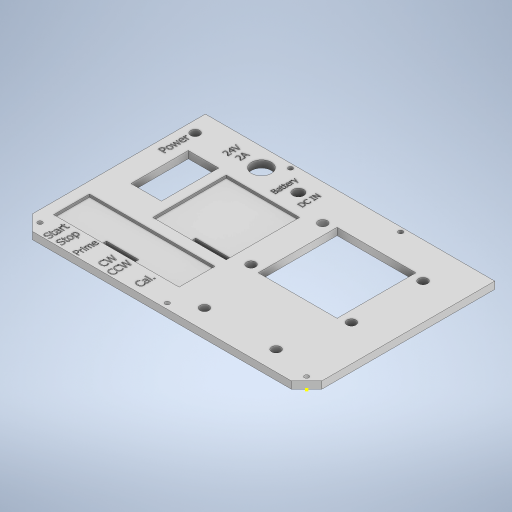
# Autodesk Inventor part: Ele Panel
Saved by Autodesk Inventor 2023 (Build 270158000, 158)
## iProperties
Created: 2023-08-23
Part Number: Ele Panel
Material: Generic
Document SubType Name: Modeling
Designer: alian
Density: 1 g/cm^3
Appearance: Default
Author: alian
Autodesk Inventor part; units mm, degrees
(part 1 of 2)
ref_plane "YZ Plane" through (0, 0, 0) normal (1, 0, 0) x (0, 1, 0)
ref_plane "XZ Plane" through (0, 0, 0) normal (0, 1, 0) x (-1, 0, 0)
ref_plane "XY Plane" through (0, 0, 0) normal (0, 0, 1) x (1, 0, 0)
sketch "Sketch1" plane through (0, 0, 0) normal (0, 1, 0) x (-1, 0, 0)
  line L0 (0, 0) -> (161.5, 0)
  line L1 (161.5, 0) -> (161.5, -105)
  line L2 (161.5, -105) -> (0, -105)
  line L3 (0, -105) -> (0, 0)
  dimension "d0" = 161.5
  dimension "d1" = 105
  constraints: 8 end point, 2 parallel, 1 horizontal, 1 perpendicular
  measures "d0" distance of L1.end L2.end
  measures "d1" distance of L0.end L1.end
extrude "Extrusion1" add sketch "Sketch1" along normal blind 4
sketch "Sketch2" plane through (0, 4, 0) normal (0, 1, 0) x (1, 0, 0)
  line L0 (-148.6423, 50.601) -> (-131.6423, 50.601)
  line L1 (-131.6423, 50.601) -> (-131.6423, 82.601)
  line L2 (-131.6423, 82.601) -> (-148.6423, 82.601)
  line L3 (-148.6423, 82.601) -> (-148.6423, 50.601)
  circle A0 centre (-148.9719, 88.0693) radius 1.5
  circle A1 centre (-131.2982, 88.0693) radius 1.5
  circle A2 centre (-131.2982, 42.7853) radius 1.5
  circle A3 centre (-148.9719, 42.7853) radius 1.5
  line L4 (-141.2539, 141.0846) -> (-141.2539, 196.4251) construction
  line L5 (-141.2539, 196.4251) -> (-113.1686, 196.4251) construction
  line L6 (-113.1686, 196.4251) -> (-113.1686, 141.0846) construction
  line L7 (-113.1686, 141.0846) -> (-141.2539, 141.0846) construction
  line L8 (-173.7219, 134.419) -> (-150.8919, 134.419)
  line L9 (-150.8919, 134.419) -> (-150.8919, 185.551)
  line L10 (-150.8919, 185.551) -> (-173.7219, 185.551)
  line L11 (-173.7219, 185.551) -> (-173.7219, 134.419)
  line L12 (-155.1907, 14) -> (-85.1907, 14)
  line L13 (-85.1907, 14) -> (-85.1907, 34)
  line L14 (-85.1907, 34) -> (-155.1907, 34)
  line L15 (-155.1907, 34) -> (-155.1907, 14)
  line L16 (-126.1907, 40.3041) -> (-85.1907, 40.3041)
  line L17 (-85.1907, 40.3041) -> (-85.1907, 81.3041)
  line L18 (-85.1907, 81.3041) -> (-126.1907, 81.3041)
  line L19 (-126.1907, 81.3041) -> (-126.1907, 40.3041)
  line L20 (-84, 33) -> (-12, 33)
  line L21 (-12, 33) -> (-12, 100)
  line L22 (-12, 100) -> (-84, 100)
  line L23 (-84, 100) -> (-84, 33)
  circle A4 centre (-68, 11) radius 2.5
  circle A5 centre (-28, 11) radius 2.5
  circle A6 centre (-119.8496, 94.6341) radius 5.5
  circle A7 centre (-97.5813, 93) radius 3
  circle A8 centre (-155.1907, 93) radius 2.5
  circle A9 centre (-88.5813, 93) radius 2.55
  line L24 (0, 105) -> (-161.5, 105) projected
  line L25 (0, 0) -> (0, 105) projected
  line L26 (-161.5, 0) -> (0, 0) projected
  line L27 (-70, 43) -> (-26, 43)
  line L28 (-26, 43) -> (-26, 87)
  line L29 (-26, 87) -> (-70, 87)
  line L30 (-70, 87) -> (-70, 43)
  point P0 (-120.1907, 14)
  point P1 (-48, 43)
  dimension "d4" = 17
  dimension "d5" = 32
  dimension "d12" = 22.83
  dimension "d13" = 51.132
  dimension "d30" = 3
  dimension "d39" = 7.8157
  dimension "d40" = 0.3296
  dimension "d42" = 0.344
  dimension "d44" = 5.4682
  dimension "d47" = 70
  dimension "d48" = 20
  dimension "d50" = 41
  dimension "d51" = 41
  dimension "d53" = 72
  dimension "d54" = 67
  dimension "d56" = 5
  dimension "d57" = 5
  dimension "d58" = 16
  dimension "d59" = 16
  dimension "d60" = 22
  dimension "d68" = 11
  dimension "d71" = 6
  dimension "d74" = 5
  dimension "d75" = 5.1
  dimension "d76" = 9
  dimension "d132" = 5
  dimension "d133" = 12
  dimension "d155" = 12
  dimension "d156" = 14
  dimension "d157" = 44
  dimension "d158" = 44
  dimension "d159" = 14
  dimension "d161" = 10
  constraints: 48 end point, 12 parallel, 10 centre point, 6 horizontal, 6 perpendicular, 5 horizontal alignment, 3 equal radius, 3 vertical alignment, 2 midpoint, 2 other
  measures "d4" distance of L2.end L1.end
  measures "d5" distance of L1.end L0.end
  measures "d12" distance of L10.end L9.end
  measures "d13" distance of L9.end L8.end
  measures "d30" diameter of A0
  measures "d39" distance from line of L0 A3.centre
  measures "d40" distance from line of A3.centre L3
  measures "d42" distance from line of L1 A2.centre
  measures "d44" distance from line of A0.centre L2
  measures "d47" distance of L14.end L13.end
  measures "d48" distance of L13.end L12.end
  measures "d50" distance of L18.end L17.end
  measures "d51" distance of L17.end L16.end
  measures "d53" distance of L22.end L21.end
  measures "d54" distance of L21.end L20.end
  measures "d56" diameter of A4
  measures "d57" diameter of A5
  measures "d58" distance from line of L23 A4.centre
  measures "d59" distance from line of L21 A5.centre
  measures "d60" distance from line of L20 A4.centre
  measures "d68" diameter of A6
  measures "d71" diameter of A7
  measures "d74" diameter of A8
  measures "d75" diameter of A9
  measures "d76" distance of A7.centre A9.centre
  measures "d132" distance between parallel lines of L24 L22
  measures "d133" distance between parallel lines of L21 L25
  measures "d155" distance from line of L24 A7.centre
  measures "d156" distance from line of L26 point (-120.191, 14)
  measures "d157" distance from line of L29 point (-48, 43)
  measures "d158" distance between parallel lines of L28 L30
  measures "d159" distance between parallel lines of L23 L30
  measures "d161" distance between parallel lines of L20 L27
extrude "Extrusion2" cut sketch "Sketch2" against normal blind 4 contours L3 L2 L1 L0 | A4 | A5 | A6 | A7 | A8 | L30 L29 L28 L27
sketch "Sketch3" plane through (0, 4, 0) normal (0, 1, 0) x (1, 0, 0)
  line L0 (-106.2715, 85.6469) -> (-106.2715, 98.9463) construction
  line L1 (-106.2715, 98.9463) -> (-102.5043, 98.9463) construction
  line L2 (-102.5043, 98.9463) -> (-102.5043, 85.6469) construction
  line L3 (-102.5043, 85.6469) -> (-106.2715, 85.6469) construction
  line L4 (-92.3295, 86.7189) -> (-92.3295, 97.75) construction
  line L5 (-92.3295, 97.75) -> (-89.0807, 97.75) construction
  line L6 (-89.0807, 97.75) -> (-89.0807, 86.7189) construction
  line L7 (-89.0807, 86.7189) -> (-92.3295, 86.7189) construction
  line L8 (-138.4009, 85.1047) -> (-138.4009, 104.5309) construction
  line L9 (-138.4009, 104.5309) -> (-128.5308, 104.5309) construction
  line L10 (-128.5308, 104.5309) -> (-128.5308, 85.1047) construction
  line L11 (-128.5308, 85.1047) -> (-138.4009, 85.1047) construction
  line L12 (-148.6469, 2.1995) -> (-148.6469, 11.1409) construction
  line L13 (-148.6469, 11.1409) -> (-144.6208, 11.1409) construction
  line L14 (-144.6208, 11.1409) -> (-144.6208, 2.1995) construction
  line L15 (-144.6208, 2.1995) -> (-148.6469, 2.1995) construction
  line L16 (-132.0468, 0.8832) -> (-132.0468, 11.3907) construction
  line L17 (-132.0468, 11.3907) -> (-128.9272, 11.3907) construction
  line L18 (-128.9272, 11.3907) -> (-128.9272, 0.8832) construction
  line L19 (-128.9272, 0.8832) -> (-132.0468, 0.8832) construction
  line L20 (-119.8791, 2.3194) -> (-119.8791, 11.1324) construction
  line L21 (-119.8791, 11.1324) -> (-111.7039, 11.1324) construction
  line L22 (-111.7039, 11.1324) -> (-111.7039, 2.3194) construction
  line L23 (-111.7039, 2.3194) -> (-119.8791, 2.3194) construction
  line L24 (-100.0402, 3.0337) -> (-100.0402, 9.9794) construction
  line L25 (-100.0402, 9.9794) -> (-92.1934, 9.9794) construction
  line L26 (-92.1934, 9.9794) -> (-92.1934, 3.0337) construction
  line L27 (-92.1934, 3.0337) -> (-100.0402, 3.0337) construction
  line L28 (-157.8178, 74.3524) -> (-157.8178, 89.3313) construction
  line L29 (-157.8178, 89.3313) -> (-153.7335, 89.3313) construction
  line L30 (-153.7335, 89.3313) -> (-153.7335, 74.3524) construction
  line L31 (-153.7335, 74.3524) -> (-157.8178, 74.3524) construction
  spline S0 degree 2 poles (-95.7906, 5.0013) (-95.7906, 4.6123) (-96.0532, 3.9543) (-96.3158, 3.7144) knots 0 0 0 1 2 2 2
  spline S1 degree 2 poles (-96.3158, 3.7144) (-96.5751, 3.4745) (-97.353, 3.212) (-97.8587, 3.212) knots 0 0 0 1 2 2 2
  spline S2 degree 2 poles (-97.8587, 3.212) (-98.3611, 3.212) (-99.1067, 3.4681) (-99.3822, 3.7112) knots 0 0 0 1 2 2 2
  spline S3 degree 2 poles (-99.3822, 3.7112) (-99.6513, 3.951) (-99.9333, 4.6058) (-99.9333, 5.011) knots 0 0 0 1 2 2 2
  spline S4 degree 2 poles (-99.9333, 5.011) (-99.9333, 5.212) (-99.8749, 5.5653) (-99.8295, 5.7144) knots 0 0 0 1 2 2 2
  spline S5 degree 2 poles (-99.8295, 5.7144) (-99.7874, 5.8441) (-99.6675, 6.1131) (-99.5962, 6.246) knots 0 0 0 1 2 2 2
  line L32 (-99.5962, 6.246) -> (-98.9543, 6.246)
  line L33 (-98.9543, 6.246) -> (-98.9543, 6.2039)
  spline S6 degree 2 poles (-98.9543, 6.2039) (-99.0192, 6.1326) (-99.2007, 5.9121) (-99.2882, 5.7533) knots 0 0 0 1 2 2 2
  spline S7 degree 2 poles (-99.2882, 5.7533) (-99.3725, 5.601) (-99.4795, 5.2412) (-99.4795, 5.0078) knots 0 0 0 1 2 2 2
  spline S8 degree 2 poles (-99.4795, 5.0078) (-99.4795, 4.7517) (-99.2688, 4.2946) (-99.0678, 4.1228) knots 0 0 0 1 2 2 2
  spline S9 degree 2 poles (-99.0678, 4.1228) (-98.8636, 3.9543) (-98.2445, 3.7663) (-97.8587, 3.7663) knots 0 0 0 1 2 2 2
  spline S10 degree 2 poles (-97.8587, 3.7663) (-97.447, 3.7663) (-96.8539, 3.964) (-96.6496, 4.1358) knots 0 0 0 1 2 2 2
  spline S11 degree 2 poles (-96.6496, 4.1358) (-96.4519, 4.3044) (-96.2509, 4.7549) (-96.2509, 5.0078) knots 0 0 0 1 2 2 2
  spline S12 degree 2 poles (-96.2509, 5.0078) (-96.2509, 5.2379) (-96.3644, 5.6301) (-96.4487, 5.7825) knots 0 0 0 1 2 2 2
  spline S13 degree 2 poles (-96.4487, 5.7825) (-96.5329, 5.9283) (-96.708, 6.1455) (-96.7696, 6.2071) knots 0 0 0 1 2 2 2
  line L34 (-96.7696, 6.2071) -> (-96.7696, 6.246)
  line L35 (-96.7696, 6.246) -> (-96.1342, 6.246)
  spline S14 degree 2 poles (-96.1342, 6.246) (-96.0727, 6.1131) (-95.9592, 5.8797) (-95.9073, 5.7144) knots 0 0 0 1 2 2 2
  spline S15 degree 2 poles (-95.9073, 5.7144) (-95.849, 5.5394) (-95.7906, 5.2412) (-95.7906, 5.0013) knots 0 0 0 1 2 2 2
  spline S16 degree 2 poles (-96.1796, 8.3757) (-96.1342, 8.3141) (-95.9722, 8.1066) (-95.9235, 8.0094) knots 0 0 0 1 2 2 2
  spline S17 degree 2 poles (-95.9235, 8.0094) (-95.8522, 7.8765) (-95.7777, 7.6269) (-95.7777, 7.4) knots 0 0 0 1 2 2 2
  spline S18 degree 2 poles (-95.7777, 7.4) (-95.7777, 7.2152) (-95.9171, 6.8813) (-96.0435, 6.7549) knots 0 0 0 1 2 2 2
  spline S19 degree 2 poles (-96.0435, 6.7549) (-96.1667, 6.635) (-96.5297, 6.4891) (-96.7307, 6.4891) knots 0 0 0 1 2 2 2
  spline S20 degree 2 poles (-96.7307, 6.4891) (-97.0419, 6.4891) (-97.4827, 6.7517) (-97.6091, 7.0369) knots 0 0 0 1 2 2 2
  spline S21 degree 2 poles (-97.6091, 7.0369) (-97.7258, 7.2898) (-97.8133, 7.977) (-97.836, 8.3757) knots 0 0 0 1 2 2 2
  line L36 (-97.836, 8.3757) -> (-97.9333, 8.3757)
  spline S22 degree 2 poles (-97.9333, 8.3757) (-98.1083, 8.3757) (-98.3255, 8.2687) (-98.3871, 8.1715) knots 0 0 0 1 2 2 2
  spline S23 degree 2 poles (-98.3871, 8.1715) (-98.4487, 8.0742) (-98.4876, 7.7954) (-98.4876, 7.6463) knots 0 0 0 1 2 2 2
  spline S24 degree 2 poles (-98.4876, 7.6463) (-98.4876, 7.4713) (-98.3838, 6.998) (-98.2833, 6.7614) knots 0 0 0 1 2 2 2
  line L37 (-98.2833, 6.7614) -> (-98.2833, 6.7322)
  line L38 (-98.2833, 6.7322) -> (-98.7987, 6.7322)
  spline S25 degree 2 poles (-98.7987, 6.7322) (-98.8376, 6.8716) (-98.9349, 7.3935) (-98.9349, 7.6496) knots 0 0 0 1 2 2 2
  spline S26 degree 2 poles (-98.9349, 7.6496) (-98.9349, 7.9608) (-98.8376, 8.3854) (-98.7112, 8.554) knots 0 0 0 1 2 2 2
  spline S27 degree 2 poles (-98.7112, 8.554) (-98.588, 8.7193) (-98.1958, 8.8813) (-97.9138, 8.8813) knots 0 0 0 1 2 2 2
  line L39 (-97.9138, 8.8813) -> (-95.862, 8.8813)
  line L40 (-95.862, 8.8813) -> (-95.862, 8.3757)
  line L41 (-95.862, 8.3757) -> (-96.1796, 8.3757)
  line L42 (-96.601, 8.3757) -> (-97.4341, 8.3757)
  spline S28 degree 2 poles (-97.4341, 8.3757) (-97.4179, 8.1942) (-97.3628, 7.6463) (-97.3109, 7.4745) knots 0 0 0 1 2 2 2
  spline S29 degree 2 poles (-97.3109, 7.4745) (-97.2493, 7.2736) (-96.9932, 7.011) (-96.7663, 7.011) knots 0 0 0 1 2 2 2
  spline S30 degree 2 poles (-96.7663, 7.011) (-96.507, 7.011) (-96.2445, 7.3027) (-96.2445, 7.5815) knots 0 0 0 1 2 2 2
  spline S31 degree 2 poles (-96.2445, 7.5815) (-96.2445, 7.8181) (-96.4487, 8.2071) (-96.601, 8.3757) knots 0 0 0 1 2 2 2
  line L43 (-95.862, 10.1066) -> (-95.862, 9.601)
  line L44 (-95.862, 9.601) -> (-100.0402, 9.601)
  line L45 (-100.0402, 9.601) -> (-100.0402, 10.1066)
  line L46 (-100.0402, 10.1066) -> (-95.862, 10.1066)
  line L47 (-95.862, 11.6334) -> (-95.862, 10.9916)
  line L48 (-95.862, 10.9916) -> (-96.6269, 10.9916)
  line L49 (-96.6269, 10.9916) -> (-96.6269, 11.6334)
  line L50 (-96.6269, 11.6334) -> (-95.862, 11.6334)
  spline S32 degree 2 poles (-115.7364, 4.5622) (-115.7364, 4.1732) (-115.999, 3.5152) (-116.2616, 3.2753) knots 0 0 0 1 2 2 2
  spline S33 degree 2 poles (-116.2616, 3.2753) (-116.5209, 3.0354) (-117.2988, 2.7729) (-117.8045, 2.7729) knots 0 0 0 1 2 2 2
  spline S34 degree 2 poles (-117.8045, 2.7729) (-118.3069, 2.7729) (-119.0525, 3.029) (-119.328, 3.2721) knots 0 0 0 1 2 2 2
  spline S35 degree 2 poles (-119.328, 3.2721) (-119.5971, 3.5119) (-119.8791, 4.1667) (-119.8791, 4.5719) knots 0 0 0 1 2 2 2
  spline S36 degree 2 poles (-119.8791, 4.5719) (-119.8791, 4.7729) (-119.8207, 5.1262) (-119.7753, 5.2753) knots 0 0 0 1 2 2 2
  spline S37 degree 2 poles (-119.7753, 5.2753) (-119.7332, 5.405) (-119.6133, 5.674) (-119.542, 5.8069) knots 0 0 0 1 2 2 2
  line L51 (-119.542, 5.8069) -> (-118.9001, 5.8069)
  line L52 (-118.9001, 5.8069) -> (-118.9001, 5.7648)
  spline S38 degree 2 poles (-118.9001, 5.7648) (-118.965, 5.6935) (-119.1465, 5.473) (-119.234, 5.3142) knots 0 0 0 1 2 2 2
  spline S39 degree 2 poles (-119.234, 5.3142) (-119.3183, 5.1619) (-119.4253, 4.8021) (-119.4253, 4.5687) knots 0 0 0 1 2 2 2
  spline S40 degree 2 poles (-119.4253, 4.5687) (-119.4253, 4.3126) (-119.2146, 3.8555) (-119.0136, 3.6837) knots 0 0 0 1 2 2 2
  spline S41 degree 2 poles (-119.0136, 3.6837) (-118.8094, 3.5152) (-118.1902, 3.3272) (-117.8045, 3.3272) knots 0 0 0 1 2 2 2
  spline S42 degree 2 poles (-117.8045, 3.3272) (-117.3928, 3.3272) (-116.7996, 3.5249) (-116.5954, 3.6967) knots 0 0 0 1 2 2 2
  spline S43 degree 2 poles (-116.5954, 3.6967) (-116.3977, 3.8653) (-116.1967, 4.3158) (-116.1967, 4.5687) knots 0 0 0 1 2 2 2
  spline S44 degree 2 poles (-116.1967, 4.5687) (-116.1967, 4.7988) (-116.3102, 5.191) (-116.3945, 5.3434) knots 0 0 0 1 2 2 2
  spline S45 degree 2 poles (-116.3945, 5.3434) (-116.4787, 5.4893) (-116.6538, 5.7064) (-116.7154, 5.768) knots 0 0 0 1 2 2 2
  line L53 (-116.7154, 5.768) -> (-116.7154, 5.8069)
  line L54 (-116.7154, 5.8069) -> (-116.08, 5.8069)
  spline S46 degree 2 poles (-116.08, 5.8069) (-116.0184, 5.674) (-115.905, 5.4406) (-115.8531, 5.2753) knots 0 0 0 1 2 2 2
  spline S47 degree 2 poles (-115.8531, 5.2753) (-115.7948, 5.1003) (-115.7364, 4.8021) (-115.7364, 4.5622) knots 0 0 0 1 2 2 2
  line L55 (-119.8078, 10.7858) -> (-115.8078, 9.781)
  line L56 (-115.8078, 9.781) -> (-115.8078, 9.1846)
  line L57 (-115.8078, 9.1846) -> (-119.127, 8.3709)
  line L58 (-119.127, 8.3709) -> (-115.8078, 7.58)
  line L59 (-115.8078, 7.58) -> (-115.8078, 6.9901)
  line L60 (-115.8078, 6.9901) -> (-119.8078, 5.969)
  line L61 (-119.8078, 5.969) -> (-119.8078, 6.5168)
  line L62 (-119.8078, 6.5168) -> (-116.4917, 7.3207)
  line L63 (-116.4917, 7.3207) -> (-119.8078, 8.1181)
  line L64 (-119.8078, 8.1181) -> (-119.8078, 8.6594)
  line L65 (-119.8078, 8.6594) -> (-116.4528, 9.4633)
  line L66 (-116.4528, 9.4633) -> (-119.8078, 10.264)
  line L67 (-119.8078, 10.264) -> (-119.8078, 10.7858)
  spline S48 degree 2 poles (-109.1505, 2.9106) (-109.1505, 2.5217) (-109.4131, 1.8636) (-109.6757, 1.6238) knots 0 0 0 1 2 2 2
  spline S49 degree 2 poles (-109.6757, 1.6238) (-109.935, 1.3839) (-110.7129, 1.1213) (-111.2186, 1.1213) knots 0 0 0 1 2 2 2
  spline S50 degree 2 poles (-111.2186, 1.1213) (-111.721, 1.1213) (-112.4666, 1.3774) (-112.7421, 1.6205) knots 0 0 0 1 2 2 2
  spline S51 degree 2 poles (-112.7421, 1.6205) (-113.0112, 1.8604) (-113.2932, 2.5152) (-113.2932, 2.9204) knots 0 0 0 1 2 2 2
  spline S52 degree 2 poles (-113.2932, 2.9204) (-113.2932, 3.1213) (-113.2348, 3.4747) (-113.1894, 3.6238) knots 0 0 0 1 2 2 2
  spline S53 degree 2 poles (-113.1894, 3.6238) (-113.1473, 3.7534) (-113.0274, 4.0225) (-112.9561, 4.1554) knots 0 0 0 1 2 2 2
  line L68 (-112.9561, 4.1554) -> (-112.3142, 4.1554)
  line L69 (-112.3142, 4.1554) -> (-112.3142, 4.1132)
  spline S54 degree 2 poles (-112.3142, 4.1132) (-112.3791, 4.0419) (-112.5606, 3.8215) (-112.6481, 3.6627) knots 0 0 0 1 2 2 2
  spline S55 degree 2 poles (-112.6481, 3.6627) (-112.7324, 3.5103) (-112.8394, 3.1505) (-112.8394, 2.9171) knots 0 0 0 1 2 2 2
  spline S56 degree 2 poles (-112.8394, 2.9171) (-112.8394, 2.6611) (-112.6287, 2.204) (-112.4277, 2.0322) knots 0 0 0 1 2 2 2
  spline S57 degree 2 poles (-112.4277, 2.0322) (-112.2235, 1.8636) (-111.6044, 1.6756) (-111.2186, 1.6756) knots 0 0 0 1 2 2 2
  spline S58 degree 2 poles (-111.2186, 1.6756) (-110.8069, 1.6756) (-110.2138, 1.8734) (-110.0095, 2.0452) knots 0 0 0 1 2 2 2
  spline S59 degree 2 poles (-110.0095, 2.0452) (-109.8118, 2.2137) (-109.6108, 2.6643) (-109.6108, 2.9171) knots 0 0 0 1 2 2 2
  spline S60 degree 2 poles (-109.6108, 2.9171) (-109.6108, 3.1473) (-109.7243, 3.5395) (-109.8086, 3.6918) knots 0 0 0 1 2 2 2
  spline S61 degree 2 poles (-109.8086, 3.6918) (-109.8928, 3.8377) (-110.0679, 4.0549) (-110.1295, 4.1165) knots 0 0 0 1 2 2 2
  line L70 (-110.1295, 4.1165) -> (-110.1295, 4.1554)
  line L71 (-110.1295, 4.1554) -> (-109.4941, 4.1554)
  spline S62 degree 2 poles (-109.4941, 4.1554) (-109.4326, 4.0225) (-109.3191, 3.7891) (-109.2672, 3.6238) knots 0 0 0 1 2 2 2
  spline S63 degree 2 poles (-109.2672, 3.6238) (-109.2089, 3.4487) (-109.1505, 3.1505) (-109.1505, 2.9106) knots 0 0 0 1 2 2 2
  spline S64 degree 2 poles (-109.1505, 6.2137) (-109.1505, 5.8247) (-109.4131, 5.1667) (-109.6757, 4.9269) knots 0 0 0 1 2 2 2
  spline S65 degree 2 poles (-109.6757, 4.9269) (-109.935, 4.687) (-110.7129, 4.4244) (-111.2186, 4.4244) knots 0 0 0 1 2 2 2
  spline S66 degree 2 poles (-111.2186, 4.4244) (-111.721, 4.4244) (-112.4666, 4.6805) (-112.7421, 4.9236) knots 0 0 0 1 2 2 2
  spline S67 degree 2 poles (-112.7421, 4.9236) (-113.0112, 5.1635) (-113.2932, 5.8183) (-113.2932, 6.2234) knots 0 0 0 1 2 2 2
  spline S68 degree 2 poles (-113.2932, 6.2234) (-113.2932, 6.4244) (-113.2348, 6.7777) (-113.1894, 6.9269) knots 0 0 0 1 2 2 2
  spline S69 degree 2 poles (-113.1894, 6.9269) (-113.1473, 7.0565) (-113.0274, 7.3256) (-112.9561, 7.4585) knots 0 0 0 1 2 2 2
  line L72 (-112.9561, 7.4585) -> (-112.3142, 7.4585)
  line L73 (-112.3142, 7.4585) -> (-112.3142, 7.4163)
  spline S70 degree 2 poles (-112.3142, 7.4163) (-112.3791, 7.345) (-112.5606, 7.1246) (-112.6481, 6.9658) knots 0 0 0 1 2 2 2
  spline S71 degree 2 poles (-112.6481, 6.9658) (-112.7324, 6.8134) (-112.8394, 6.4536) (-112.8394, 6.2202) knots 0 0 0 1 2 2 2
  spline S72 degree 2 poles (-112.8394, 6.2202) (-112.8394, 5.9641) (-112.6287, 5.5071) (-112.4277, 5.3353) knots 0 0 0 1 2 2 2
  spline S73 degree 2 poles (-112.4277, 5.3353) (-112.2235, 5.1667) (-111.6044, 4.9787) (-111.2186, 4.9787) knots 0 0 0 1 2 2 2
  spline S74 degree 2 poles (-111.2186, 4.9787) (-110.8069, 4.9787) (-110.2138, 5.1764) (-110.0095, 5.3482) knots 0 0 0 1 2 2 2
  spline S75 degree 2 poles (-110.0095, 5.3482) (-109.8118, 5.5168) (-109.6108, 5.9674) (-109.6108, 6.2202) knots 0 0 0 1 2 2 2
  spline S76 degree 2 poles (-109.6108, 6.2202) (-109.6108, 6.4504) (-109.7243, 6.8426) (-109.8086, 6.9949) knots 0 0 0 1 2 2 2
  spline S77 degree 2 poles (-109.8086, 6.9949) (-109.8928, 7.1408) (-110.0679, 7.358) (-110.1295, 7.4196) knots 0 0 0 1 2 2 2
  line L74 (-110.1295, 7.4196) -> (-110.1295, 7.4585)
  line L75 (-110.1295, 7.4585) -> (-109.4941, 7.4585)
  spline S78 degree 2 poles (-109.4941, 7.4585) (-109.4326, 7.3256) (-109.3191, 7.0922) (-109.2672, 6.9269) knots 0 0 0 1 2 2 2
  spline S79 degree 2 poles (-109.2672, 6.9269) (-109.2089, 6.7518) (-109.1505, 6.4536) (-109.1505, 6.2137) knots 0 0 0 1 2 2 2
  line L76 (-113.2219, 12.4374) -> (-109.2219, 11.4325)
  line L77 (-109.2219, 11.4325) -> (-109.2219, 10.8361)
  line L78 (-109.2219, 10.8361) -> (-112.5411, 10.0225)
  line L79 (-112.5411, 10.0225) -> (-109.2219, 9.2316)
  line L80 (-109.2219, 9.2316) -> (-109.2219, 8.6416)
  line L81 (-109.2219, 8.6416) -> (-113.2219, 7.6205)
  line L82 (-113.2219, 7.6205) -> (-113.2219, 8.1683)
  line L83 (-113.2219, 8.1683) -> (-109.9058, 8.9722)
  line L84 (-109.9058, 8.9722) -> (-113.2219, 9.7696)
  line L85 (-113.2219, 9.7696) -> (-113.2219, 10.311)
  line L86 (-113.2219, 10.311) -> (-109.8669, 11.1149)
  line L87 (-109.8669, 11.1149) -> (-113.2219, 11.9155)
  line L88 (-113.2219, 11.9155) -> (-113.2219, 12.4374)
  spline S80 degree 2 poles (-130.969, 3.4501) (-130.7421, 3.4501) (-130.3337, 3.2884) (-130.1919, 3.1437) knots 0 0 0 1 2 2 2
  spline S81 degree 2 poles (-130.1919, 3.1437) (-130.0132, 2.9622) (-129.8288, 2.4715) (-129.8288, 2.0972) knots 0 0 0 1 2 2 2
  line L89 (-129.8288, 2.0972) -> (-129.8288, 1.7029)
  line L90 (-129.8288, 1.7029) -> (-128.5241, 1.7029)
  line L91 (-128.5241, 1.7029) -> (-128.5241, 1.2378)
  line L92 (-128.5241, 1.2378) -> (-132.0241, 1.2378)
  line L93 (-132.0241, 1.2378) -> (-132.0241, 2.117)
  spline S82 degree 2 poles (-132.0241, 2.117) (-132.0241, 2.429) (-131.922, 2.8658) (-131.8057, 3.0331) knots 0 0 0 1 2 2 2
  spline S83 degree 2 poles (-131.8057, 3.0331) (-131.6724, 3.2288) (-131.2612, 3.4501) (-130.969, 3.4501) knots 0 0 0 1 2 2 2
  spline S84 degree 2 poles (-130.9549, 2.9651) (-131.1364, 2.9651) (-131.403, 2.8403) (-131.4881, 2.7126) knots 0 0 0 1 2 2 2
  spline S85 degree 2 poles (-131.4881, 2.7126) (-131.5618, 2.602) (-131.6214, 2.307) (-131.6214, 2.0886) knots 0 0 0 1 2 2 2
  line L94 (-131.6214, 2.0886) -> (-131.6214, 1.7029)
  line L95 (-131.6214, 1.7029) -> (-130.2259, 1.7029)
  line L96 (-130.2259, 1.7029) -> (-130.2259, 2.0206)
  spline S86 degree 2 poles (-130.2259, 2.0206) (-130.2259, 2.3042) (-130.3167, 2.6531) (-130.4358, 2.7665) knots 0 0 0 1 2 2 2
  spline S87 degree 2 poles (-130.4358, 2.7665) (-130.5408, 2.8715) (-130.7875, 2.9651) (-130.9549, 2.9651) knots 0 0 0 1 2 2 2
  line L97 (-130.6769, 5.2511) -> (-130.6769, 5.2284)
  spline S88 degree 2 poles (-130.6769, 5.2284) (-130.6911, 5.1774) (-130.6968, 5.0668) (-130.6968, 4.9902) knots 0 0 0 1 2 2 2
  spline S89 degree 2 poles (-130.6968, 4.9902) (-130.6968, 4.8115) (-130.5408, 4.4598) (-130.3876, 4.301) knots 0 0 0 1 2 2 2
  line L98 (-130.3876, 4.301) -> (-128.5241, 4.301)
  line L99 (-128.5241, 4.301) -> (-128.5241, 3.8585)
  line L100 (-128.5241, 3.8585) -> (-131.1506, 3.8585)
  line L101 (-131.1506, 3.8585) -> (-131.1506, 4.301)
  line L102 (-131.1506, 4.301) -> (-130.7592, 4.301)
  spline S90 degree 2 poles (-130.7592, 4.301) (-130.9747, 4.542) (-131.1506, 4.9023) (-131.1506, 5.0724) knots 0 0 0 1 2 2 2
  spline S91 degree 2 poles (-131.1506, 5.0724) (-131.1506, 5.1405) (-131.1449, 5.2086) (-131.1364, 5.2511) knots 0 0 0 1 2 2 2
  line L103 (-131.1364, 5.2511) -> (-130.6769, 5.2511)
  line L104 (-128.5241, 6.0453) -> (-128.5241, 5.6028)
  line L105 (-128.5241, 5.6028) -> (-131.1506, 5.6028)
  line L106 (-131.1506, 5.6028) -> (-131.1506, 6.0453)
  line L107 (-131.1506, 6.0453) -> (-128.5241, 6.0453)
  line L108 (-131.5874, 6.0765) -> (-131.5874, 5.5745)
  line L109 (-131.5874, 5.5745) -> (-132.0468, 5.5745)
  line L110 (-132.0468, 5.5745) -> (-132.0468, 6.0765)
  line L111 (-132.0468, 6.0765) -> (-131.5874, 6.0765)
  line L112 (-128.5241, 9.6729) -> (-130.0444, 9.6729)
  spline S92 degree 2 poles (-130.0444, 9.6729) (-130.2259, 9.6729) (-130.5351, 9.6446) (-130.6202, 9.5992) knots 0 0 0 1 2 2 2
  spline S93 degree 2 poles (-130.6202, 9.5992) (-130.7138, 9.5538) (-130.8045, 9.3808) (-130.8045, 9.2305) knots 0 0 0 1 2 2 2
  spline S94 degree 2 poles (-130.8045, 9.2305) (-130.8045, 9.0943) (-130.6372, 8.7823) (-130.4784, 8.6178) knots 0 0 0 1 2 2 2
  spline S95 degree 2 poles (-130.4784, 8.6178) (-130.4386, 8.6207) (-130.328, 8.6263) (-130.2543, 8.6263) knots 0 0 0 1 2 2 2
  line L113 (-130.2543, 8.6263) -> (-128.5241, 8.6263)
  line L114 (-128.5241, 8.6263) -> (-128.5241, 8.1839)
  line L115 (-128.5241, 8.1839) -> (-130.0444, 8.1839)
  spline S96 degree 2 poles (-130.0444, 8.1839) (-130.2259, 8.1839) (-130.5351, 8.1555) (-130.6202, 8.1101) knots 0 0 0 1 2 2 2
  spline S97 degree 2 poles (-130.6202, 8.1101) (-130.7138, 8.0647) (-130.8045, 7.8917) (-130.8045, 7.7414) knots 0 0 0 1 2 2 2
  spline S98 degree 2 poles (-130.8045, 7.7414) (-130.8045, 7.5996) (-130.6258, 7.2848) (-130.4869, 7.1373) knots 0 0 0 1 2 2 2
  line L116 (-130.4869, 7.1373) -> (-128.5241, 7.1373)
  line L117 (-128.5241, 7.1373) -> (-128.5241, 6.6948)
  line L118 (-128.5241, 6.6948) -> (-131.1506, 6.6948)
  line L119 (-131.1506, 6.6948) -> (-131.1506, 7.1373)
  line L120 (-131.1506, 7.1373) -> (-130.8613, 7.1373)
  spline S99 degree 2 poles (-130.8613, 7.1373) (-131.0343, 7.3103) (-131.2243, 7.6506) (-131.2243, 7.8549) knots 0 0 0 1 2 2 2
  spline S100 degree 2 poles (-131.2243, 7.8549) (-131.2243, 8.0874) (-131.0116, 8.4476) (-130.7705, 8.5412) knots 0 0 0 1 2 2 2
  spline S101 degree 2 poles (-130.7705, 8.5412) (-130.9946, 8.7426) (-131.2243, 9.1227) (-131.2243, 9.3439) knots 0 0 0 1 2 2 2
  spline S102 degree 2 poles (-131.2243, 9.3439) (-131.2243, 9.5141) (-131.1194, 9.792) (-131.0002, 9.8942) knots 0 0 0 1 2 2 2
  spline S103 degree 2 poles (-131.0002, 9.8942) (-130.8811, 9.9991) (-130.5237, 10.1154) (-130.2543, 10.1154) knots 0 0 0 1 2 2 2
  line L121 (-130.2543, 10.1154) -> (-128.5241, 10.1154)
  line L122 (-128.5241, 10.1154) -> (-128.5241, 9.6729)
  spline S104 degree 2 poles (-128.4646, 11.8767) (-128.4646, 11.2471) (-129.1708, 10.555) (-129.8232, 10.555) knots 0 0 0 1 2 2 2
  spline S105 degree 2 poles (-129.8232, 10.555) (-130.4642, 10.555) (-131.2243, 11.2272) (-131.2243, 11.769) knots 0 0 0 1 2 2 2
  spline S106 degree 2 poles (-131.2243, 11.769) (-131.2243, 12.0129) (-131.0825, 12.3901) (-130.9322, 12.5291) knots 0 0 0 1 2 2 2
  spline S107 degree 2 poles (-130.9322, 12.5291) (-130.7818, 12.6709) (-130.3479, 12.8212) (-130.0331, 12.8212) knots 0 0 0 1 2 2 2
  line L123 (-130.0331, 12.8212) -> (-129.792, 12.8212)
  line L124 (-129.792, 12.8212) -> (-129.792, 11.0031)
  spline S108 degree 2 poles (-129.792, 11.0031) (-129.3353, 11.0031) (-128.8503, 11.4626) (-128.8503, 11.8711) knots 0 0 0 1 2 2 2
  spline S109 degree 2 poles (-128.8503, 11.8711) (-128.8503, 12.0157) (-128.9156, 12.2965) (-128.9666, 12.41) knots 0 0 0 1 2 2 2
  spline S110 degree 2 poles (-128.9666, 12.41) (-129.0233, 12.5291) (-129.1226, 12.6936) (-129.168, 12.7475) knots 0 0 0 1 2 2 2
  line L125 (-129.168, 12.7475) -> (-129.168, 12.773)
  line L126 (-129.168, 12.773) -> (-128.6858, 12.773)
  spline S111 degree 2 poles (-128.6858, 12.773) (-128.6546, 12.6964) (-128.5639, 12.4638) (-128.5383, 12.3731) knots 0 0 0 1 2 2 2
  spline S112 degree 2 poles (-128.5383, 12.3731) (-128.5015, 12.2454) (-128.4646, 12.0356) (-128.4646, 11.8767) knots 0 0 0 1 2 2 2
  spline S113 degree 2 poles (-130.1295, 12.3901) (-130.3082, 12.3844) (-130.5691, 12.3107) (-130.657, 12.2398) knots 0 0 0 1 2 2 2
  spline S114 degree 2 poles (-130.657, 12.2398) (-130.7563, 12.1632) (-130.8613, 11.9221) (-130.8613, 11.7434) knots 0 0 0 1 2 2 2
  spline S115 degree 2 poles (-130.8613, 11.7434) (-130.8613, 11.5676) (-130.7563, 11.3208) (-130.6542, 11.2187) knots 0 0 0 1 2 2 2
  spline S116 degree 2 poles (-130.6542, 11.2187) (-130.5493, 11.1194) (-130.2968, 11.0173) (-130.1295, 11.0031) knots 0 0 0 1 2 2 2
  line L127 (-130.1295, 11.0031) -> (-130.1295, 12.3901)
  spline S117 degree 2 poles (-144.5043, 2.3817) (-144.5043, 1.9473) (-144.6858, 1.3379) (-144.8155, 1.0689) knots 0 0 0 1 2 2 2
  line L128 (-144.8155, 1.0689) -> (-145.4832, 1.0689)
  line L129 (-145.4832, 1.0689) -> (-145.4832, 1.1078)
  spline S118 degree 2 poles (-145.4832, 1.1078) (-145.2368, 1.3703) (-144.9646, 2.0349) (-144.9646, 2.3428) knots 0 0 0 1 2 2 2
  spline S119 degree 2 poles (-144.9646, 2.3428) (-144.9646, 2.7836) (-145.3309, 3.2342) (-145.6323, 3.2342) knots 0 0 0 1 2 2 2
  spline S120 degree 2 poles (-145.6323, 3.2342) (-145.8722, 3.2342) (-146.1704, 2.9976) (-146.245, 2.7415) knots 0 0 0 1 2 2 2
  spline S121 degree 2 poles (-146.245, 2.7415) (-146.2968, 2.5567) (-146.3681, 2.2488) (-146.4265, 2.0186) knots 0 0 0 1 2 2 2
  spline S122 degree 2 poles (-146.4265, 2.0186) (-146.4816, 1.8112) (-146.6469, 1.4838) (-146.7798, 1.3574) knots 0 0 0 1 2 2 2
  spline S123 degree 2 poles (-146.7798, 1.3574) (-146.9127, 1.2342) (-147.2693, 1.0981) (-147.5027, 1.0981) knots 0 0 0 1 2 2 2
  spline S124 degree 2 poles (-147.5027, 1.0981) (-147.9889, 1.0981) (-148.6469, 1.8566) (-148.6469, 2.4433) knots 0 0 0 1 2 2 2
  spline S125 degree 2 poles (-148.6469, 2.4433) (-148.6469, 2.7804) (-148.514, 3.3768) (-148.3876, 3.6329) knots 0 0 0 1 2 2 2
  line L130 (-148.3876, 3.6329) -> (-147.7522, 3.6329)
  line L131 (-147.7522, 3.6329) -> (-147.7522, 3.594)
  spline S126 degree 2 poles (-147.7522, 3.594) (-147.9273, 3.4028) (-148.1866, 2.8063) (-148.1866, 2.4789) knots 0 0 0 1 2 2 2
  spline S127 degree 2 poles (-148.1866, 2.4789) (-148.1866, 2.1094) (-147.8398, 1.6524) (-147.5578, 1.6524) knots 0 0 0 1 2 2 2
  spline S128 degree 2 poles (-147.5578, 1.6524) (-147.3049, 1.6524) (-147.0035, 1.9214) (-146.9354, 2.1742) knots 0 0 0 1 2 2 2
  spline S129 degree 2 poles (-146.9354, 2.1742) (-146.89, 2.3428) (-146.7733, 2.8323) (-146.7247, 2.9943) knots 0 0 0 1 2 2 2
  spline S130 degree 2 poles (-146.7247, 2.9943) (-146.5983, 3.406) (-146.0894, 3.7885) (-145.7166, 3.7885) knots 0 0 0 1 2 2 2
  spline S131 degree 2 poles (-145.7166, 3.7885) (-145.48, 3.7885) (-145.0262, 3.5973) (-144.8673, 3.4255) knots 0 0 0 1 2 2 2
  spline S132 degree 2 poles (-144.8673, 3.4255) (-144.6923, 3.2342) (-144.5043, 2.748) (-144.5043, 2.3817) knots 0 0 0 1 2 2 2
  spline S133 degree 2 poles (-144.5172, 5.1985) (-144.5172, 4.7869) (-144.9873, 4.3233) (-145.4962, 4.3233) knots 0 0 0 1 2 2 2
  line L132 (-145.4962, 4.3233) -> (-147.1591, 4.3233)
  line L133 (-147.1591, 4.3233) -> (-147.1591, 3.983)
  line L134 (-147.1591, 3.983) -> (-147.5772, 3.983)
  line L135 (-147.5772, 3.983) -> (-147.5772, 4.3233)
  line L136 (-147.5772, 4.3233) -> (-148.4394, 4.3233)
  line L137 (-148.4394, 4.3233) -> (-148.4394, 4.829)
  line L138 (-148.4394, 4.829) -> (-147.5772, 4.829)
  line L139 (-147.5772, 4.829) -> (-147.5772, 5.7593)
  line L140 (-147.5772, 5.7593) -> (-147.1591, 5.7593)
  line L141 (-147.1591, 5.7593) -> (-147.1591, 4.829)
  line L142 (-147.1591, 4.829) -> (-145.7296, 4.829)
  spline S134 degree 2 poles (-145.7296, 4.829) (-145.5027, 4.829) (-145.2531, 4.8452) (-145.1461, 4.9003) knots 0 0 0 1 2 2 2
  spline S135 degree 2 poles (-145.1461, 4.9003) (-145.0521, 4.9457) (-144.9581, 5.1499) (-144.9581, 5.325) knots 0 0 0 1 2 2 2
  spline S136 degree 2 poles (-144.9581, 5.325) (-144.9581, 5.4481) (-145.0326, 5.6783) (-145.0553, 5.7302) knots 0 0 0 1 2 2 2
  line L143 (-145.0553, 5.7302) -> (-145.0553, 5.7593)
  line L144 (-145.0553, 5.7593) -> (-144.6015, 5.7593)
  spline S137 degree 2 poles (-144.6015, 5.7593) (-144.5626, 5.6167) (-144.5172, 5.325) (-144.5172, 5.1985) knots 0 0 0 1 2 2 2
  spline S138 degree 2 poles (-144.8932, 7.8047) (-144.8479, 7.7431) (-144.6858, 7.5357) (-144.6372, 7.4384) knots 0 0 0 1 2 2 2
  spline S139 degree 2 poles (-144.6372, 7.4384) (-144.5659, 7.3055) (-144.4913, 7.0559) (-144.4913, 6.829) knots 0 0 0 1 2 2 2
  spline S140 degree 2 poles (-144.4913, 6.829) (-144.4913, 6.6443) (-144.6307, 6.3104) (-144.7571, 6.184) knots 0 0 0 1 2 2 2
  spline S141 degree 2 poles (-144.7571, 6.184) (-144.8803, 6.064) (-145.2433, 5.9182) (-145.4443, 5.9182) knots 0 0 0 1 2 2 2
  spline S142 degree 2 poles (-145.4443, 5.9182) (-145.7555, 5.9182) (-146.1963, 6.1807) (-146.3227, 6.466) knots 0 0 0 1 2 2 2
  spline S143 degree 2 poles (-146.3227, 6.466) (-146.4394, 6.7188) (-146.527, 7.406) (-146.5497, 7.8047) knots 0 0 0 1 2 2 2
  line L145 (-146.5497, 7.8047) -> (-146.6469, 7.8047)
  spline S144 degree 2 poles (-146.6469, 7.8047) (-146.8219, 7.8047) (-147.0391, 7.6977) (-147.1007, 7.6005) knots 0 0 0 1 2 2 2
  spline S145 degree 2 poles (-147.1007, 7.6005) (-147.1623, 7.5032) (-147.2012, 7.2245) (-147.2012, 7.0754) knots 0 0 0 1 2 2 2
  spline S146 degree 2 poles (-147.2012, 7.0754) (-147.2012, 6.9003) (-147.0975, 6.4271) (-146.997, 6.1904) knots 0 0 0 1 2 2 2
  line L146 (-146.997, 6.1904) -> (-146.997, 6.1613)
  line L147 (-146.997, 6.1613) -> (-147.5124, 6.1613)
  spline S147 degree 2 poles (-147.5124, 6.1613) (-147.5513, 6.3007) (-147.6485, 6.8225) (-147.6485, 7.0786) knots 0 0 0 1 2 2 2
  spline S148 degree 2 poles (-147.6485, 7.0786) (-147.6485, 7.3898) (-147.5513, 7.8144) (-147.4249, 7.983) knots 0 0 0 1 2 2 2
  spline S149 degree 2 poles (-147.4249, 7.983) (-147.3017, 8.1483) (-146.9095, 8.3104) (-146.6274, 8.3104) knots 0 0 0 1 2 2 2
  line L148 (-146.6274, 8.3104) -> (-144.5756, 8.3104)
  line L149 (-144.5756, 8.3104) -> (-144.5756, 7.8047)
  line L150 (-144.5756, 7.8047) -> (-144.8932, 7.8047)
  line L151 (-145.3146, 7.8047) -> (-146.1477, 7.8047)
  spline S150 degree 2 poles (-146.1477, 7.8047) (-146.1315, 7.6232) (-146.0764, 7.0754) (-146.0245, 6.9036) knots 0 0 0 1 2 2 2
  spline S151 degree 2 poles (-146.0245, 6.9036) (-145.9629, 6.7026) (-145.7069, 6.44) (-145.48, 6.44) knots 0 0 0 1 2 2 2
  spline S152 degree 2 poles (-145.48, 6.44) (-145.2206, 6.44) (-144.9581, 6.7318) (-144.9581, 7.0105) knots 0 0 0 1 2 2 2
  spline S153 degree 2 poles (-144.9581, 7.0105) (-144.9581, 7.2472) (-145.1623, 7.6362) (-145.3146, 7.8047) knots 0 0 0 1 2 2 2
  line L152 (-147.0359, 10.6118) -> (-147.0359, 10.5859)
  spline S154 degree 2 poles (-147.0359, 10.5859) (-147.0521, 10.5276) (-147.0586, 10.4011) (-147.0586, 10.3136) knots 0 0 0 1 2 2 2
  spline S155 degree 2 poles (-147.0586, 10.3136) (-147.0586, 10.1094) (-146.8803, 9.7075) (-146.7052, 9.5259) knots 0 0 0 1 2 2 2
  line L153 (-146.7052, 9.5259) -> (-144.5756, 9.5259)
  line L154 (-144.5756, 9.5259) -> (-144.5756, 9.0203)
  line L155 (-144.5756, 9.0203) -> (-147.5772, 9.0203)
  line L156 (-147.5772, 9.0203) -> (-147.5772, 9.5259)
  line L157 (-147.5772, 9.5259) -> (-147.1299, 9.5259)
  spline S156 degree 2 poles (-147.1299, 9.5259) (-147.3762, 9.8015) (-147.5772, 10.2131) (-147.5772, 10.4076) knots 0 0 0 1 2 2 2
  spline S157 degree 2 poles (-147.5772, 10.4076) (-147.5772, 10.4854) (-147.5707, 10.5632) (-147.561, 10.6118) knots 0 0 0 1 2 2 2
  line L158 (-147.561, 10.6118) -> (-147.0359, 10.6118)
  spline S158 degree 2 poles (-144.5172, 11.9117) (-144.5172, 11.5) (-144.9873, 11.0365) (-145.4962, 11.0365) knots 0 0 0 1 2 2 2
  line L159 (-145.4962, 11.0365) -> (-147.1591, 11.0365)
  line L160 (-147.1591, 11.0365) -> (-147.1591, 10.6961)
  line L161 (-147.1591, 10.6961) -> (-147.5772, 10.6961)
  line L162 (-147.5772, 10.6961) -> (-147.5772, 11.0365)
  line L163 (-147.5772, 11.0365) -> (-148.4394, 11.0365)
  line L164 (-148.4394, 11.0365) -> (-148.4394, 11.5421)
  line L165 (-148.4394, 11.5421) -> (-147.5772, 11.5421)
  line L166 (-147.5772, 11.5421) -> (-147.5772, 12.4725)
  line L167 (-147.5772, 12.4725) -> (-147.1591, 12.4725)
  line L168 (-147.1591, 12.4725) -> (-147.1591, 11.5421)
  line L169 (-147.1591, 11.5421) -> (-145.7296, 11.5421)
  spline S159 degree 2 poles (-145.7296, 11.5421) (-145.5027, 11.5421) (-145.2531, 11.5584) (-145.1461, 11.6135) knots 0 0 0 1 2 2 2
  spline S160 degree 2 poles (-145.1461, 11.6135) (-145.0521, 11.6588) (-144.9581, 11.8631) (-144.9581, 12.0381) knots 0 0 0 1 2 2 2
  spline S161 degree 2 poles (-144.9581, 12.0381) (-144.9581, 12.1613) (-145.0326, 12.3914) (-145.0553, 12.4433) knots 0 0 0 1 2 2 2
  line L170 (-145.0553, 12.4433) -> (-145.0553, 12.4725)
  line L171 (-145.0553, 12.4725) -> (-144.6015, 12.4725)
  spline S162 degree 2 poles (-144.6015, 12.4725) (-144.5626, 12.3298) (-144.5172, 12.0381) (-144.5172, 11.9117) knots 0 0 0 1 2 2 2
  spline S163 degree 2 poles (-137.9184, 2.7253) (-137.9184, 2.2909) (-138.0999, 1.6815) (-138.2296, 1.4125) knots 0 0 0 1 2 2 2
  line L172 (-138.2296, 1.4125) -> (-138.8973, 1.4125)
  line L173 (-138.8973, 1.4125) -> (-138.8973, 1.4514)
  spline S164 degree 2 poles (-138.8973, 1.4514) (-138.651, 1.7139) (-138.3787, 2.3785) (-138.3787, 2.6864) knots 0 0 0 1 2 2 2
  spline S165 degree 2 poles (-138.3787, 2.6864) (-138.3787, 3.1272) (-138.745, 3.5778) (-139.0464, 3.5778) knots 0 0 0 1 2 2 2
  spline S166 degree 2 poles (-139.0464, 3.5778) (-139.2863, 3.5778) (-139.5845, 3.3412) (-139.6591, 3.0851) knots 0 0 0 1 2 2 2
  spline S167 degree 2 poles (-139.6591, 3.0851) (-139.7109, 2.9003) (-139.7822, 2.5924) (-139.8406, 2.3622) knots 0 0 0 1 2 2 2
  spline S168 degree 2 poles (-139.8406, 2.3622) (-139.8957, 2.1548) (-140.061, 1.8274) (-140.1939, 1.701) knots 0 0 0 1 2 2 2
  spline S169 degree 2 poles (-140.1939, 1.701) (-140.3268, 1.5778) (-140.6834, 1.4417) (-140.9168, 1.4417) knots 0 0 0 1 2 2 2
  spline S170 degree 2 poles (-140.9168, 1.4417) (-141.403, 1.4417) (-142.061, 2.2002) (-142.061, 2.7869) knots 0 0 0 1 2 2 2
  spline S171 degree 2 poles (-142.061, 2.7869) (-142.061, 3.124) (-141.9281, 3.7204) (-141.8017, 3.9765) knots 0 0 0 1 2 2 2
  line L174 (-141.8017, 3.9765) -> (-141.1664, 3.9765)
  line L175 (-141.1664, 3.9765) -> (-141.1664, 3.9376)
  spline S172 degree 2 poles (-141.1664, 3.9376) (-141.3414, 3.7464) (-141.6007, 3.1499) (-141.6007, 2.8225) knots 0 0 0 1 2 2 2
  spline S173 degree 2 poles (-141.6007, 2.8225) (-141.6007, 2.453) (-141.2539, 1.996) (-140.9719, 1.996) knots 0 0 0 1 2 2 2
  spline S174 degree 2 poles (-140.9719, 1.996) (-140.719, 1.996) (-140.4176, 2.265) (-140.3495, 2.5178) knots 0 0 0 1 2 2 2
  spline S175 degree 2 poles (-140.3495, 2.5178) (-140.3041, 2.6864) (-140.1874, 3.1759) (-140.1388, 3.3379) knots 0 0 0 1 2 2 2
  spline S176 degree 2 poles (-140.1388, 3.3379) (-140.0124, 3.7496) (-139.5035, 4.1321) (-139.1307, 4.1321) knots 0 0 0 1 2 2 2
  spline S177 degree 2 poles (-139.1307, 4.1321) (-138.8941, 4.1321) (-138.4403, 3.9409) (-138.2814, 3.7691) knots 0 0 0 1 2 2 2
  spline S178 degree 2 poles (-138.2814, 3.7691) (-138.1064, 3.5778) (-137.9184, 3.0916) (-137.9184, 2.7253) knots 0 0 0 1 2 2 2
  spline S179 degree 2 poles (-137.9313, 5.5421) (-137.9313, 5.1305) (-138.4014, 4.6669) (-138.9103, 4.6669) knots 0 0 0 1 2 2 2
  line L176 (-138.9103, 4.6669) -> (-140.5732, 4.6669)
  line L177 (-140.5732, 4.6669) -> (-140.5732, 4.3266)
  line L178 (-140.5732, 4.3266) -> (-140.9913, 4.3266)
  line L179 (-140.9913, 4.3266) -> (-140.9913, 4.6669)
  line L180 (-140.9913, 4.6669) -> (-141.8535, 4.6669)
  line L181 (-141.8535, 4.6669) -> (-141.8535, 5.1726)
  line L182 (-141.8535, 5.1726) -> (-140.9913, 5.1726)
  line L183 (-140.9913, 5.1726) -> (-140.9913, 6.1029)
  line L184 (-140.9913, 6.1029) -> (-140.5732, 6.1029)
  line L185 (-140.5732, 6.1029) -> (-140.5732, 5.1726)
  line L186 (-140.5732, 5.1726) -> (-139.1437, 5.1726)
  spline S180 degree 2 poles (-139.1437, 5.1726) (-138.9168, 5.1726) (-138.6672, 5.1888) (-138.5602, 5.2439) knots 0 0 0 1 2 2 2
  spline S181 degree 2 poles (-138.5602, 5.2439) (-138.4662, 5.2893) (-138.3722, 5.4935) (-138.3722, 5.6686) knots 0 0 0 1 2 2 2
  spline S182 degree 2 poles (-138.3722, 5.6686) (-138.3722, 5.7917) (-138.4467, 6.0219) (-138.4694, 6.0738) knots 0 0 0 1 2 2 2
  line L187 (-138.4694, 6.0738) -> (-138.4694, 6.1029)
  line L188 (-138.4694, 6.1029) -> (-138.0156, 6.1029)
  spline S183 degree 2 poles (-138.0156, 6.1029) (-137.9767, 5.9603) (-137.9313, 5.6686) (-137.9313, 5.5421) knots 0 0 0 1 2 2 2
  spline S184 degree 2 poles (-139.4905, 8.9425) (-138.732, 8.9425) (-137.9054, 8.2131) (-137.9054, 7.6037) knots 0 0 0 1 2 2 2
  spline S185 degree 2 poles (-137.9054, 7.6037) (-137.9054, 6.9781) (-138.7579, 6.2618) (-139.4905, 6.2618) knots 0 0 0 1 2 2 2
  spline S186 degree 2 poles (-139.4905, 6.2618) (-140.2425, 6.2618) (-141.0756, 7.0008) (-141.0756, 7.6037) knots 0 0 0 1 2 2 2
  spline S187 degree 2 poles (-141.0756, 7.6037) (-141.0756, 8.2131) (-140.2458, 8.9425) (-139.4905, 8.9425) knots 0 0 0 1 2 2 2
  spline S188 degree 2 poles (-139.4905, 8.4206) (-140.074, 8.4206) (-140.6412, 7.996) (-140.6412, 7.6037) knots 0 0 0 1 2 2 2
  spline S189 degree 2 poles (-140.6412, 7.6037) (-140.6412, 7.2115) (-140.074, 6.7836) (-139.4905, 6.7836) knots 0 0 0 1 2 2 2
  spline S190 degree 2 poles (-139.4905, 6.7836) (-138.9232, 6.7836) (-138.3398, 7.2115) (-138.3398, 7.6037) knots 0 0 0 1 2 2 2
  spline S191 degree 2 poles (-138.3398, 7.6037) (-138.3398, 7.9927) (-138.9135, 8.4206) (-139.4905, 8.4206) knots 0 0 0 1 2 2 2
  spline S192 degree 2 poles (-139.5715, 11.9765) (-138.8195, 11.9765) (-137.9313, 11.2601) (-137.9313, 10.7123) knots 0 0 0 1 2 2 2
  spline S193 degree 2 poles (-137.9313, 10.7123) (-137.9313, 10.4887) (-138.0351, 10.1451) (-138.142, 9.9668) knots 0 0 0 1 2 2 2
  line L189 (-138.142, 9.9668) -> (-136.8843, 9.9668)
  line L190 (-136.8843, 9.9668) -> (-136.8843, 9.4611)
  line L191 (-136.8843, 9.4611) -> (-140.9913, 9.4611)
  line L192 (-140.9913, 9.4611) -> (-140.9913, 9.9668)
  line L193 (-140.9913, 9.9668) -> (-140.6769, 9.9668)
  spline S194 degree 2 poles (-140.6769, 9.9668) (-140.8487, 10.1548) (-141.0756, 10.6151) (-141.0756, 10.8841) knots 0 0 0 1 2 2 2
  spline S195 degree 2 poles (-141.0756, 10.8841) (-141.0756, 11.3995) (-140.2587, 11.9765) (-139.5715, 11.9765) knots 0 0 0 1 2 2 2
  spline S196 degree 2 poles (-139.5132, 11.4546) (-140.0286, 11.4546) (-140.5958, 11.1272) (-140.5958, 10.7609) knots 0 0 0 1 2 2 2
  spline S197 degree 2 poles (-140.5958, 10.7609) (-140.5958, 10.547) (-140.4046, 10.1451) (-140.2555, 9.9668) knots 0 0 0 1 2 2 2
  line L194 (-140.2555, 9.9668) -> (-138.5505, 9.9668)
  spline S198 degree 2 poles (-138.5505, 9.9668) (-138.4565, 10.1645) (-138.3852, 10.4465) (-138.3852, 10.628) knots 0 0 0 1 2 2 2
  spline S199 degree 2 poles (-138.3852, 10.628) (-138.3852, 11.0203) (-138.9621, 11.4546) (-139.5132, 11.4546) knots 0 0 0 1 2 2 2
  line L195 (-134.8272, 93.1486) -> (-134.8272, 90.9902)
  line L196 (-134.8272, 90.9902) -> (-135.3236, 90.9902)
  spline S200 degree 2 poles (-135.3236, 90.9902) (-135.542, 91.2228) (-135.9475, 91.6369) (-136.1659, 91.8354) knots 0 0 0 1 2 2 2
  spline S201 degree 2 poles (-136.1659, 91.8354) (-136.6056, 92.2353) (-137.1331, 92.5275) (-137.4139, 92.5275) knots 0 0 0 1 2 2 2
  spline S202 degree 2 poles (-137.4139, 92.5275) (-137.5614, 92.5275) (-137.7826, 92.4367) (-137.8535, 92.3545) knots 0 0 0 1 2 2 2
  spline S203 degree 2 poles (-137.8535, 92.3545) (-137.9244, 92.2722) (-137.9954, 92.0567) (-137.9954, 91.9262) knots 0 0 0 1 2 2 2
  spline S204 degree 2 poles (-137.9954, 91.9262) (-137.9954, 91.8014) (-137.933, 91.5461) (-137.8847, 91.4298) knots 0 0 0 1 2 2 2
  spline S205 degree 2 poles (-137.8847, 91.4298) (-137.845, 91.3306) (-137.7316, 91.1462) (-137.6919, 91.0895) knots 0 0 0 1 2 2 2
  line L197 (-137.6919, 91.0895) -> (-137.6919, 91.064)
  line L198 (-137.6919, 91.064) -> (-138.1911, 91.064)
  spline S206 degree 2 poles (-138.1911, 91.064) (-138.262, 91.2086) (-138.4009, 91.7276) (-138.4009, 91.9602) knots 0 0 0 1 2 2 2
  spline S207 degree 2 poles (-138.4009, 91.9602) (-138.4009, 92.4509) (-137.8819, 93.004) (-137.4394, 93.004) knots 0 0 0 1 2 2 2
  spline S208 degree 2 poles (-137.4394, 93.004) (-137.2324, 93.004) (-136.8864, 92.9076) (-136.7389, 92.8225) knots 0 0 0 1 2 2 2
  spline S209 degree 2 poles (-136.7389, 92.8225) (-136.5857, 92.7374) (-136.2851, 92.4906) (-136.1404, 92.3545) knots 0 0 0 1 2 2 2
  spline S210 degree 2 poles (-136.1404, 92.3545) (-135.8993, 92.1332) (-135.3831, 91.5915) (-135.2328, 91.4298) knots 0 0 0 1 2 2 2
  line L199 (-135.2328, 91.4298) -> (-135.2328, 93.1486)
  line L200 (-135.2328, 93.1486) -> (-134.8272, 93.1486)
  line L201 (-136.0298, 95.8687) -> (-136.0298, 95.4517)
  line L202 (-136.0298, 95.4517) -> (-134.8272, 95.4517)
  line L203 (-134.8272, 95.4517) -> (-134.8272, 95.0007)
  line L204 (-134.8272, 95.0007) -> (-136.0298, 95.0007)
  line L205 (-136.0298, 95.0007) -> (-136.0298, 93.455)
  line L206 (-136.0298, 93.455) -> (-136.5233, 93.455)
  line L207 (-136.5233, 93.455) -> (-138.3272, 95.0206)
  line L208 (-138.3272, 95.0206) -> (-138.3272, 95.4517)
  line L209 (-138.3272, 95.4517) -> (-136.407, 95.4517)
  line L210 (-136.407, 95.4517) -> (-136.407, 95.8687)
  line L211 (-136.407, 95.8687) -> (-136.0298, 95.8687)
  line L212 (-136.407, 95.0007) -> (-137.7741, 95.0007)
  line L213 (-137.7741, 95.0007) -> (-136.407, 93.8237)
  line L214 (-136.407, 93.8237) -> (-136.407, 95.0007)
  line L215 (-138.3272, 98.8808) -> (-134.8272, 97.6754)
  line L216 (-134.8272, 97.6754) -> (-134.8272, 97.1734)
  line L217 (-134.8272, 97.1734) -> (-138.3272, 95.9679)
  line L218 (-138.3272, 95.9679) -> (-138.3272, 96.4671)
  line L219 (-138.3272, 96.4671) -> (-135.42, 97.4371)
  line L220 (-135.42, 97.4371) -> (-138.3272, 98.4071)
  line L221 (-138.3272, 98.4071) -> (-138.3272, 98.8808)
  line L222 (-129.0645, 94.4519) -> (-129.0645, 92.2935)
  line L223 (-129.0645, 92.2935) -> (-129.5609, 92.2935)
  spline S211 degree 2 poles (-129.5609, 92.2935) (-129.7793, 92.5261) (-130.1849, 92.9402) (-130.4033, 93.1387) knots 0 0 0 1 2 2 2
  spline S212 degree 2 poles (-130.4033, 93.1387) (-130.8429, 93.5386) (-131.3705, 93.8308) (-131.6513, 93.8308) knots 0 0 0 1 2 2 2
  spline S213 degree 2 poles (-131.6513, 93.8308) (-131.7987, 93.8308) (-132.02, 93.74) (-132.0909, 93.6578) knots 0 0 0 1 2 2 2
  spline S214 degree 2 poles (-132.0909, 93.6578) (-132.1618, 93.5755) (-132.2327, 93.3599) (-132.2327, 93.2295) knots 0 0 0 1 2 2 2
  spline S215 degree 2 poles (-132.2327, 93.2295) (-132.2327, 93.1047) (-132.1703, 92.8494) (-132.1221, 92.7331) knots 0 0 0 1 2 2 2
  spline S216 degree 2 poles (-132.1221, 92.7331) (-132.0824, 92.6338) (-131.9689, 92.4495) (-131.9292, 92.3928) knots 0 0 0 1 2 2 2
  line L224 (-131.9292, 92.3928) -> (-131.9292, 92.3672)
  line L225 (-131.9292, 92.3672) -> (-132.4284, 92.3672)
  spline S217 degree 2 poles (-132.4284, 92.3672) (-132.4993, 92.5119) (-132.6383, 93.0309) (-132.6383, 93.2635) knots 0 0 0 1 2 2 2
  spline S218 degree 2 poles (-132.6383, 93.2635) (-132.6383, 93.7542) (-132.1192, 94.3073) (-131.6768, 94.3073) knots 0 0 0 1 2 2 2
  spline S219 degree 2 poles (-131.6768, 94.3073) (-131.4697, 94.3073) (-131.1237, 94.2108) (-130.9762, 94.1257) knots 0 0 0 1 2 2 2
  spline S220 degree 2 poles (-130.9762, 94.1257) (-130.8231, 94.0407) (-130.5224, 93.7939) (-130.3778, 93.6578) knots 0 0 0 1 2 2 2
  spline S221 degree 2 poles (-130.3778, 93.6578) (-130.1367, 93.4365) (-129.6205, 92.8948) (-129.4701, 92.7331) knots 0 0 0 1 2 2 2
  line L226 (-129.4701, 92.7331) -> (-129.4701, 94.4519)
  line L227 (-129.4701, 94.4519) -> (-129.0645, 94.4519)
  line L228 (-129.0645, 94.642) -> (-132.5645, 95.8219)
  line L229 (-132.5645, 95.8219) -> (-132.5645, 96.3948)
  line L230 (-132.5645, 96.3948) -> (-129.0645, 97.5747)
  line L231 (-129.0645, 97.5747) -> (-129.0645, 97.084)
  line L232 (-129.0645, 97.084) -> (-130.0431, 96.7663)
  line L233 (-130.0431, 96.7663) -> (-130.0431, 95.4304)
  line L234 (-130.0431, 95.4304) -> (-129.0645, 95.1128)
  line L235 (-129.0645, 95.1128) -> (-129.0645, 94.642)
  line L236 (-130.4402, 96.6387) -> (-132.088, 96.097)
  line L237 (-132.088, 96.097) -> (-130.4402, 95.5581)
  line L238 (-130.4402, 95.5581) -> (-130.4402, 96.6387)
  spline S222 degree 2 poles (-104.1596, 88.023) (-103.9324, 88.023) (-103.5841, 87.8501) (-103.4705, 87.7069) knots 0 0 0 1 2 2 2
  spline S223 degree 2 poles (-103.4705, 87.7069) (-103.3371, 87.534) (-103.2235, 87.1412) (-103.2235, 86.83) knots 0 0 0 1 2 2 2
  line L239 (-103.2235, 86.83) -> (-103.2235, 85.9556)
  line L240 (-103.2235, 85.9556) -> (-106.2715, 85.9556)
  line L241 (-106.2715, 85.9556) -> (-106.2715, 86.7633)
  spline S224 degree 2 poles (-106.2715, 86.7633) (-106.2715, 87.0894) (-106.2295, 87.4154) (-106.148, 87.5636) knots 0 0 0 1 2 2 2
  spline S225 degree 2 poles (-106.148, 87.5636) (-106.0615, 87.7291) (-105.7775, 87.8798) (-105.5848, 87.8798) knots 0 0 0 1 2 2 2
  spline S226 degree 2 poles (-105.5848, 87.8798) (-105.3699, 87.8798) (-105.029, 87.6525) (-104.9327, 87.4525) knots 0 0 0 1 2 2 2
  line L242 (-104.9327, 87.4525) -> (-104.9179, 87.4525)
  spline S227 degree 2 poles (-104.9179, 87.4525) (-104.8438, 87.7242) (-104.4511, 88.023) (-104.1596, 88.023) knots 0 0 0 1 2 2 2
  spline S228 degree 2 poles (-104.1423, 87.6007) (-104.3152, 87.6007) (-104.5375, 87.5019) (-104.6166, 87.3537) knots 0 0 0 1 2 2 2
  spline S229 degree 2 poles (-104.6166, 87.3537) (-104.666, 87.2573) (-104.6956, 87.0301) (-104.6956, 86.8201) knots 0 0 0 1 2 2 2
  line L243 (-104.6956, 86.8201) -> (-104.6956, 86.3607)
  line L244 (-104.6956, 86.3607) -> (-103.5693, 86.3607)
  line L245 (-103.5693, 86.3607) -> (-103.5693, 86.6892)
  spline S230 degree 2 poles (-103.5693, 86.6892) (-103.5693, 86.956) (-103.6187, 87.2623) (-103.6977, 87.3808) knots 0 0 0 1 2 2 2
  spline S231 degree 2 poles (-103.6977, 87.3808) (-103.7792, 87.4945) (-103.9818, 87.6007) (-104.1423, 87.6007) knots 0 0 0 1 2 2 2
  spline S232 degree 2 poles (-105.528, 87.4574) (-105.6367, 87.4574) (-105.7997, 87.3833) (-105.8466, 87.3018) knots 0 0 0 1 2 2 2
  spline S233 degree 2 poles (-105.8466, 87.3018) (-105.901, 87.203) (-105.9257, 86.9634) (-105.9257, 86.7485) knots 0 0 0 1 2 2 2
  line L246 (-105.9257, 86.7485) -> (-105.9257, 86.3607)
  line L247 (-105.9257, 86.3607) -> (-105.034, 86.3607)
  line L248 (-105.034, 86.3607) -> (-105.034, 86.8201)